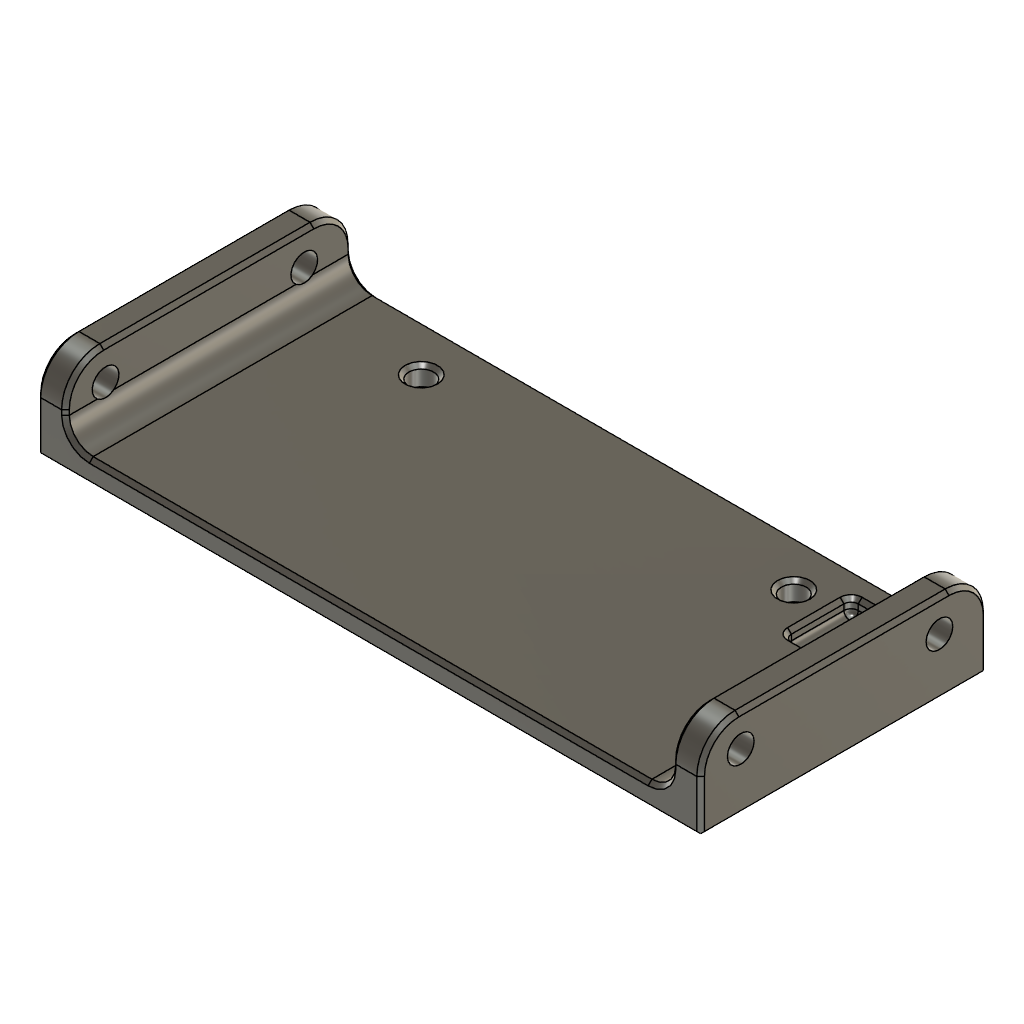
TLA704_CF_ADAPTER (Autodesk Fusion 360 design; units mm, degrees)
Autodesk Fusion 360 part; units mm, degrees
sketch "Sketch1" plane through (0, 0, 0) normal (0, 0, 1) x (1, 0, 0)
  line L0 (0, 0) -> (69.5, 0)
  line L1 (69.5, 0) -> (69.5, 30)
  line L2 (69.5, 30) -> (0, 30)
  line L3 (0, 30) -> (0, 0)
  line L4 (3, 30) -> (3, 0)
  line L5 (66.5, 30) -> (66.5, 0)
  dimension "d1" = 69.5
  dimension "d2" = 30
  dimension "d3" = 3
  dimension "d4" = 3
  constraint horizontal L0
  constraint vertical L1
  constraint horizontal L2
  constraint vertical L3
  constraint coincident L0.start L3.end
  constraint coincident L2 L4.start
  constraint coincident L0 L4.end
  constraint perpendicular L0 L4
  constraint coincident L2 L5.start
  constraint coincident L0 L5.end
  constraint perpendicular L0 L5
  measures "d1" distance of L0.start L0.end
  measures "d2" distance of L0.start L2.end
  measures "d3" distance of L3 L4
  measures "d4" distance of L1 L5
extrude "Extrude1" add sketch "Sketch1" along normal blind 2.4
extrude "Extrude2" add sketch "Sketch1" along normal blind 7 from surface at 2.4 contours L0 L2 L3 L4 | L0 L1 L2 L5
sketch "Sketch2" plane through (0, 0, 0) normal (-1, 0, 0) x (0, -1, 0)
  line L0 (-30, 0) -> (0, 0)
  line L1 (0, 0) -> (0, 9.4)
  line L2 (0, 9.4) -> (-30, 9.4)
  line L3 (-30, 9.4) -> (-30, 0)
  circle A0 centre (-4.2, 6) radius 1.4
  circle A1 centre (-25, 6) radius 1.4
  line L4 (-30, 0) -> (0, 0)
  dimension "d11" = 6
  dimension "d12" = 6
  dimension "d13" = 2.8
  dimension "d14" = 2.8
  dimension "d15" = 20.8
  dimension "d16" = 5
  measures "d11" distance of A0.centre L4
  measures "d12" distance of A1.centre L4
  measures "d13" diameter of A0
  measures "d14" diameter of A1
  measures "d15" distance of A0.centre A1.centre
  measures "d16" distance of L3 A1.centre
extrude "Extrude3" cut sketch "Sketch2" against normal up to surface (69.5 mm away) contours A0 | A1
sketch "Sketch3" plane through (0, 0, 2.4) normal (0, 0, 1) x (-1, 0, 0)
  line L0 (-66.5, 0) -> (-66.5, -30)
  line L1 (-66.5, -30) -> (-3, -30)
  line L2 (-3, -30) -> (-3, 0)
  line L3 (-3, 0) -> (-66.5, 0)
  line L4 (0, -23.6) -> (0, -26.4)
  line L5 (-3, -26.4) -> (-3, -23.6)
  line L6 (-66.5, -23.6) -> (-66.5, -26.4)
  line L7 (-69.5, -26.4) -> (-69.5, -23.6)
  line L8 (0, -25) -> (-69.5, -25) construction
  circle A0 centre (-15.25, -25) radius 1.3
  circle A1 centre (-54.25, -25) radius 1.3
  line L9 (-34.75, -30) -> (-34.75, 0) construction
  line L10 (-57.75, -27.5) -> (-60.75, -27.5)
  line L11 (-60.75, -27.5) -> (-60.75, -20.5)
  line L12 (-60.75, -20.5) -> (-57.75, -20.5)
  line L13 (-57.75, -20.5) -> (-57.75, -27.5)
  dimension "d19" = 39
  dimension "d21" = 2.6
  dimension "d22" = 2.6
  dimension "d23" = 3.5
  dimension "d24" = 6.5
  dimension "d25" = 2.5
  dimension "d26" = 4.5
  constraint midpoint L4 L8.start
  constraint midpoint L7 L8.end
  constraint coincident L8 A0.centre
  constraint coincident L8 A1.centre
  constraint midpoint L1 L9.start
  constraint midpoint L3 L9.end
  constraint symmetric A0.centre A1.centre L9
  constraint horizontal L10
  constraint vertical L11
  constraint horizontal L12
  constraint vertical L13
  measures "d19" distance of A0.centre A1.centre
  measures "d21" diameter of A0
  measures "d22" diameter of A1
  measures "d23" distance of A1.centre L13
  measures "d24" distance of A1.centre L11
  measures "d25" distance of A1.centre L10
  measures "d26" distance of A1.centre L12
extrude "Extrude4" cut sketch "Sketch3" against normal through all contours A0 | A1
extrude "Extrude5" cut sketch "Sketch3" against normal blind 1.6 contours L10 L11 L12 L13
fillet "Fillet1" radius 0.75 4 edges at (60.75, 20.5, 1.6) (57.75, 20.5, 1.6) (60.75, 27.5, 1.6) (57.75, 27.5, 1.6)
fillet "Fillet2" radius 2.5 2 edges at (66.5, 15, 2.4) (3, 15, 2.4)
chamfer "Chamfer1" distance 0.4 angle 45 16 edges at (34.75, 30, 0) (0, 15, 0) (34.75, 0, 0) (69.5, 15, 0) (55.462, 25.4701, 0) (16.462, 25.4701, 0) (16.462, 24.5299, 2.4) (55.462, 24.5299, 2.4) (57.75, 24, 2.4) (57.9697, 27.2803, 2.4) (59.25, 27.5, 2.4) (60.5303, 27.2803, 2.4) (60.75, 24, 2.4) (60.5303, 20.7197, 2.4) (59.25, 20.5, 2.4) (57.9697, 20.7197, 2.4)
fillet "Fillet3" radius 0.6 8 edges at (60.5303, 20.7197, 0.8) (59.25, 20.5, 0.8) (57.9697, 20.7197, 0.8) (57.75, 24, 0.8) (57.9697, 27.2803, 0.8) (59.25, 27.5, 0.8) (60.5303, 27.2803, 0.8) (60.75, 24, 0.8)
fillet "Fillet4" radius 4 tangency weight 1.02818 4 edges at (68, 30, 9.4) (68, 0, 9.4) (1.5, 30, 9.4) (1.5, 0, 9.4)
chamfer "Chamfer2" distance 0.4 angle 45 26 edges at (66.5, 15, 9.4) (66.5, 1.1582, 8.2421) (66.5, 0, 5.15) (65.7678, 0, 3.1322) (34.75, 0, 2.4) (3.7322, 0, 3.1322) (3, 0, 5.15) (3, 1.1579, 8.2418) (3, 15, 9.4) (3, 28.8418, 8.2421) (3, 30, 5.15) (3.7322, 30, 3.1322) (34.75, 30, 2.4) (65.7678, 30, 3.1322) (66.5, 30, 5.15) (66.5, 28.8421, 8.2418) (69.5, 15, 9.4) (69.5, 28.8418, 8.2421) (69.5, 30, 2.9) (69.5, 0, 2.9) (69.5, 1.1579, 8.2418) (0, 15, 9.4) (0, 1.1582, 8.2421) (0, 0, 2.9) (0, 30, 2.9) (0, 28.8421, 8.2418)
equation "d4 = d3"
equation "d12 = d11"
equation "d14 = d13"
equation "d22 = d21"
named bodies: "tla704_cf_adapter"
